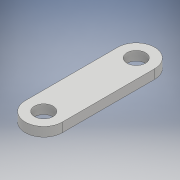
# Autodesk Inventor part: 圓盤
Saved by Autodesk Inventor 2017 (Build 210142000, 142)
## iProperties
Part Number: 圓盤
Material: 一般
Document SubType Name: Modeling
Designer: user
Density: 1 g/cm^3
Appearance: 預設
Author: user
Autodesk Inventor part; units mm, degrees
ref_plane "YZ Plane" through (0, 0, 0) normal (1, 0, 0) x (0, 1, 0)
ref_plane "XZ Plane" through (0, 0, 0) normal (0, 1, 0) x (-1, 0, 0)
ref_plane "XY Plane" through (0, 0, 0) normal (0, 0, 1) x (1, 0, 0)
sketch "草圖1" plane through (0, 0, 0) normal (0, 0, 1) x (1, 0, 0)
  line L0 (0, -5) -> (0, 5) construction
  line L1 (2, -5) -> (2, 5)
  line L2 (-2, 5) -> (-2, -5)
  arc A0 (-2, -5) -> (2, -5) centre (0, -5) ccw
  arc A1 (2, 5) -> (-2, 5) centre (0, 5) ccw
  point P0 (0, 0)
  dimension "d0" = 10
  dimension "d21" = 4
  constraints: 8 end point, 4 point on circle, 4 tangent, 2 centre point, 1 midpoint, 1 parallel, 1 vertical
  measures "d0" distance of L0.start L0.end
  measures "d21" distance between parallel lines of L1 L2
extrude "擠出1" add sketch "草圖1" along normal mid plane 1
sketch "草圖2" plane through (0, 0, 0) normal (0, 0, 1) x (1, 0, 0)
  arc A0 (-2, -5) -> (2, -5) centre (0, -5) ccw projected
  circle A1 centre (0, -5) radius 0.75
  point P0 (0, 0)
  dimension "d3" = 1.5
  constraints: 1 centre point, 1 coincident
  measures "d3" diameter of A1
extrude "擠出2" add sketch "草圖2" along normal mid plane 3
sketch "草圖3" plane through (0, 0, 0) normal (0, 0, 1) x (1, 0, 0)
  arc A0 (2, 5) -> (-2, 5) centre (0, 5) ccw projected
  circle A1 centre (0, 5) radius 0.75
  point P0 (0, 0)
  dimension "d6" = 1.5
  constraints: 1 centre point, 1 coincident
  measures "d6" diameter of A1
extrude "擠出3" add sketch "草圖3" along normal mid plane 3
sketch "草圖4" plane through (2, -5, 0.5) normal (1, 0, 0) x (0, 0, -1)
  line L0 (0, 0) -> (0, -2) projected
  line L1 (0, -2) -> (-2.346, -2)
  line L2 (-2.346, -2) -> (-2.346, 2.4059)
  line L3 (-2.346, 2.4059) -> (0, 2.4059)
  line L4 (0, 2.4059) -> (0, -2)
  point P0 (0.5, 5)
  constraints: 8 end point, 2 parallel, 1 horizontal, 1 perpendicular
extrude "擠出4" cut sketch "草圖4" against normal blind 10
sketch "草圖5" plane through (0, 0, -0.5) normal (0, 0, -1) x (-1, 0, 0)
  circle A0 centre (0, 5) radius 0.75 projected
  point P0 (0, 0)
extrude "擠出5" cut sketch "草圖5" along normal blind 10
sketch "草圖7" plane through (0, 5, 1.5) normal (0, 0, 1) x (1, 0, 0)
  circle A0 centre (0, 0) radius 0.75
  circle A1 centre (0, 0) radius 0.75 projected
  circle A2 centre (0, -10) radius 0.75 projected
  point P0 (0, -5)
  constraints: 1 centre point
extrude "擠出7" cut sketch "草圖7" against normal blind 10
sketch "草圖8" plane through (0, 0, 0.5) normal (0, 0, 1) x (1, 0, 0)
  circle A0 centre (0, 5) radius 0.75 projected
  circle A1 centre (0, 5) radius 1
  circle A2 centre (0, -5) radius 0.75 projected
  circle A3 centre (0, -5) radius 1
  point P0 (0, 0)
  dimension "d17" = 2
  dimension "d18" = 2
  constraints: 2 centre point, 2 coincident
  measures "d17" diameter of A1
  measures "d18" diameter of A3
extrude "擠出8" cut sketch "草圖8" against normal blind 10
